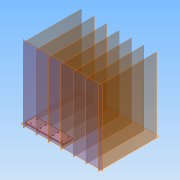
# Autodesk Inventor part: Timing_Backboard 2 Lanes
Saved by Autodesk Inventor 2018.1 (Build 221171000, 171)
## iProperties
Created: 2019-02-12
Part Number: Timing_Backboard 2 Lanes
Material: Wood (Oak)
Document SubType Name: Modeling
Designer: James
Density: 0.76 g/cm^3
Appearance: White Oak - Natural Medium Gloss
Author: James
Autodesk Inventor part; units mm, degrees
ref_plane "YZ Plane" through (0, 0, 0) normal (1, 0, 0) x (0, 1, 0)
ref_plane "XZ Plane" through (0, 0, 0) normal (0, 1, 0) x (-1, 0, 0)
ref_plane "XY Plane" through (0, 0, 0) normal (0, 0, 1) x (1, 0, 0)
derived "Selection_Skeleton.ipt"
ref_plane "Ground" through (0, 0, 0) normal (0, 1, 0) x (-1, 0, 0)
ref_plane "LHS inner" through (0, 0, 0) normal (1, 0, 0) x (0, 1, 0)
ref_plane "RHS inner" through (300, 0, 0) normal (1, 0, 0) x (0, 1, 0)
ref_plane "Lane 1" through (50, 0, 0) normal (1, 0, 0) x (0, 1, 0)
ref_plane "Lane 2" through (100, 0, 0) normal (1, 0, 0) x (0, 1, 0)
ref_plane "Lane 3" through (150, 0, 0) normal (1, 0, 0) x (0, 1, 0)
ref_plane "Lane 4" through (200, 0, 0) normal (1, 0, 0) x (0, 1, 0)
ref_plane "Lane 5" through (250, 0, 0) normal (1, 0, 0) x (0, 1, 0)
ref_plane "Back" through (0, 0, 0) normal (0, 0, 1) x (1, 0, 0)
sketch "Sketch1" plane through (0, 0, 0) normal (0, 0, 1) x (1, 0, 0)
  line L0 (0, 48) -> (0, -8) projected
  line L1 (50, 48) -> (50, -8) projected
  line L2 (100, 48) -> (100, -8) projected
  line L3 (150, 48) -> (150, -8) projected
  line L4 (200, 48) -> (200, -8) projected
  line L5 (250, 48) -> (250, -8) projected
  line L6 (-30, 0) -> (180, 0) projected
  line L7 (0, 0) -> (150, 0)
  line L8 (150, 0) -> (150, 40)
  line L9 (150, 40) -> (0, 40)
  line L10 (0, 40) -> (0, 0)
  dimension "d1" = 40
  constraints: 8 end point, 2 parallel, 1 collinear, 1 horizontal, 1 perpendicular
  measures "d1" distance of L7.end L8.end
extrude "Extrusion1" add sketch "Sketch1" along normal blind 5
sketch "Sketch2" plane through (0, 0, 0) normal (0, 0, -1) x (-1, 0, 0)
  line L0 (-50, -8) -> (-50, 48) projected
  line L1 (-150, 40) -> (0, 40) projected
  line L2 (0, 0) -> (-150, 0) projected
  point P0 (-50, 30)
  point P1 (-50, 10)
  dimension "d4" = 20
  dimension "d5" = 10
  dimension "d6" = 10
  constraints: 2 point on line
  measures "d4" distance of point (-50, 10) point (-50, 30)
  measures "d5" distance from line of L1 point (-50, 30)
  measures "d6" distance from line of L2 point (-50, 10)
hole "Hole1" at (50, 30, 0) at (50, 10, 0) direction (0, 0, 1) diameter 4.5 end through all clearance for "Socket Head Cap Screw" size "M4" standard "Ansi Metric M Profile"
pattern_linear "Rectangular Pattern1" count 2 spacing 50 along (1, 0, 0) of "Hole1"
sketch "Sketch3" plane through (0, 0, 5) normal (0, 0, 1) x (1, 0, 0)
  line L0 (0, 48) -> (0, -8) projected
  line L1 (300, 48) -> (300, -8) projected
  line L2 (150, 40) -> (0, 40) projected
  line L3 (-50, 0) -> (300, 0) projected
  line L4 (250, 48) -> (250, -8) projected
  line L5 (150, 48) -> (150, -8) projected
  point P0 (0, 0)
  point P1 (12.5, 32.5)
  point P2 (12.5, 7.5)
  point P3 (137.5, 32.5)
  point P4 (137.5, 7.5)
  dimension "d17" = 12.5
  dimension "d19" = 7.5
  dimension "d20" = 7.5
  dimension "d29" = 12.5
  constraints: 2 horizontal alignment, 2 vertical alignment, 2 other
  measures "d17" distance from line of point (12.5, 32.5) L0
  measures "d19" distance from line of L2 point (137.5, 32.5)
  measures "d20" distance from line of L3 point (137.5, 7.5)
  measures "d29" distance from line of L5 point (137.5, 32.5)
hole "Hole2" at (12.5, 32.5, 5) at (12.5, 7.5, 5) at (137.5, 32.5, 5) at (137.5, 7.5, 5) direction (0, 0, -1) diameter 4.5 end through all clearance for "Socket Head Cap Screw" size "M4" standard "Ansi Metric M Profile"
equation "\"d5\" = d6"
equation "\"d20\" = d19"
equation "\"d29\" = d17"
body "Solid1"
